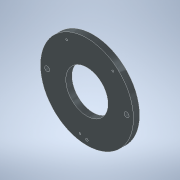
# Autodesk Inventor part: В сальник
Saved by Autodesk Inventor 2021 (Build 250183000, 183)
## iProperties
Created: 2020-12-18
Part Number: В сальник
Material: Чугун, серый
Document SubType Name: Modeling
Designer: Тимоха
Mass: 1204.61 g
Surface Area: 362.98 cm^2
Volume: 168.477 cm^3
Density: 7.15 g/cm^3
Appearance: Чугун серый
Author: Тимоха
Autodesk Inventor part; units mm, degrees
ref_plane "YZ Plane" through (0, 0, 0) normal (1, 0, 0) x (0, 1, 0)
ref_plane "XZ Plane" through (0, 0, 0) normal (0, 1, 0) x (-1, 0, 0)
ref_plane "XY Plane" through (0, 0, 0) normal (0, 0, 1) x (1, 0, 0)
sketch "Эскиз1" plane through (0, 0, 0) normal (0, 0, 1) x (1, 0, 0)
  circle A0 centre (0, 0) radius 75
  circle A1 centre (0, 0) radius 34
  dimension "d0" = 150
  dimension "d1" = 68
  constraints: 2 centre point, 2 coincident
  measures "d0" diameter of A0
  measures "d1" diameter of A1
extrude "Выдавливание1" add sketch "Эскиз1" along normal blind 10
sketch "Эскиз2" plane through (0, 0, 10) normal (0, 0, 1) x (1, 0, 0)
  circle A0 centre (-64, 0) radius 4
  point P0 (0, 0)
  dimension "d4" = 8
  dimension "d5" = 64
  constraints: 1 centre point
  measures "d4" diameter of A0
  measures "d5" distance of A0.centre point (0, 0)
extrude "Выдавливание2" cut sketch "Эскиз2" against normal blind 12
pattern_circular "Круговой массив1" count 2 over 360 about axis through (0, 0, 0) along (0, 0, 1) of "Выдавливание2"
sketch "Эскиз3" plane through (0, 0, 0) normal (0, 1, 0) x (-1, 0, 0)
  line L0 (0, 0) -> (0, 5)
  dimension "d32" = 5
  constraints: 2 end point, 1 vertical
  measures "d32" distance of L0.start L0.end
hole "Отверстие1" at (0, 0, 5) direction (0, 1, 0) diameter 4.9 depth 69 tip angle 118 counterbore diameter 5 counterbore depth 68.705
sketch "Эскиз4" plane through (0, 0, 0) normal (0, 0, -1) x (-1, 0, 0)
  circle A0 centre (0, 0) radius 34 projected
  line L0 (0, -34) -> (0, -67)
  circle A1 centre (0, -67) radius 2
  dimension "d18" = 33
  dimension "d33" = 4
  constraints: 2 end point, 1 centre point, 1 coincident, 1 vertical, 1 vertical alignment, 1 other
  measures "d18" distance of L0.start L0.end
  measures "d33" diameter of A1
extrude "Выдавливание3" cut sketch "Эскиз4" against normal blind 12 contours A1
sketch "Эскиз6" plane through (0, 0, 0) normal (0, 0, -1) x (-1, 0, 0)
  line L0 (0, 0) -> (0, 67)
  circle A0 centre (0, 67) radius 2
  dimension "d34" = 67
  dimension "d35" = 4
  constraints: 2 end point, 1 centre point, 1 coincident, 1 vertical
  measures "d34" distance of L0.start L0.end
  measures "d35" diameter of A0
extrude "Выдавливание5" cut sketch "Эскиз6" against normal blind 5
sketch "Эскиз7" plane through (0, 0, 0) normal (0, 0, -1) x (-1, 0, 0)
  circle A0 centre (64, 0) radius 4 projected
  circle A1 centre (-64, 0) radius 4 projected
  circle A2 centre (64, 0) radius 5
  circle A3 centre (-64, 0) radius 5
  point P0 (0, 0)
  dimension "d38" = 10
  dimension "d39" = 10
  constraints: 2 centre point, 2 coincident
  measures "d38" diameter of A2
  measures "d39" diameter of A3
extrude "Выдавливание6" cut sketch "Эскиз7" against normal blind 1
sketch "Эскиз8" plane through (0, 0, 0) normal (0, 0, -1) x (-1, 0, 0)
  circle A0 centre (32.5, 56.2917) radius 1.5 projected
  circle A1 centre (11.2871, -64.0125) radius 1.5 projected
  circle A2 centre (-41.7812, 49.7929) radius 1.5 projected
  point P0 (0, 0)
extrude "Выдавливание7" cut sketch "Эскиз8" against normal through all
